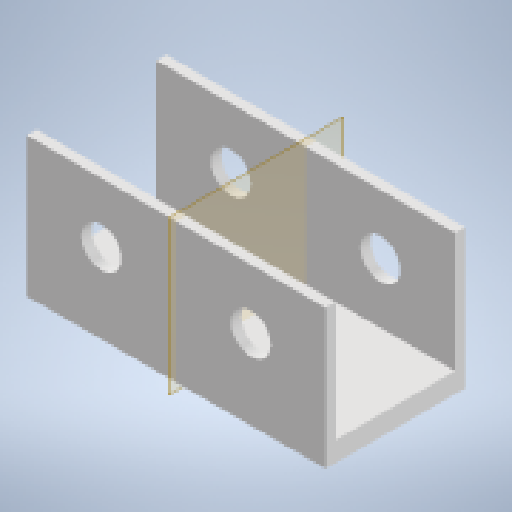
# Autodesk Inventor part: baza
Saved by Autodesk Inventor 2025 (Build 290162000, 162)
## iProperties
Created: 2025-02-05
Part Number: baza
Material: Generic
Document SubType Name: Modeling
Designer: piotr
Density: 1 g/cm^3
Appearance: Default
Author: piotr
Autodesk Inventor part; units mm, degrees
ref_plane "YZ Plane" through (0, 0, 0) normal (1, 0, 0) x (0, 1, 0)
ref_plane "XZ Plane" through (0, 0, 0) normal (0, 1, 0) x (-1, 0, 0)
ref_plane "XY Plane" through (0, 0, 0) normal (0, 0, 1) x (1, 0, 0)
sketch "Sketch1" plane through (0, 0, 0) normal (1, 0, 0) x (0, 1, 0)
  line L0 (0, 0) -> (0, -70)
  line L1 (0, 0) -> (70, 0)
  line L2 (70, 0) -> (70, -5)
  line L3 (70, -5) -> (10, -5)
  line L4 (10, -5) -> (10, -65)
  line L5 (10, -65) -> (70, -65)
  line L6 (70, -65) -> (70, -70)
  line L7 (70, -70) -> (0, -70)
  dimension "d0" = 70
  dimension "d1" = 70
  dimension "d2" = 5
  dimension "d3" = 60
  dimension "d4" = 60
  dimension "d5" = 60
  dimension "d6" = 5
  constraints: 16 end point, 3 horizontal, 3 perpendicular, 2 vertical, 1 point on line
  measures "d0" distance of L0.start L0.end
  measures "d1" distance of L0.start L1.end
  measures "d2" distance of L1.end L2.end
  measures "d3" distance of L2.end L3.end
  measures "d4" distance of L3.end L4.end
  measures "d5" distance of L4.end L5.end
  measures "d6" distance of L5.end L6.end
extrude "Extrusion1" add sketch "Sketch1" along normal blind 150
sketch "Sketch2" plane through (0, 0, 0) normal (0, 0, 1) x (1, 0, 0)
  line L0 (0, 0) -> (0, 70) projected
  line L1 (150, 70) -> (150, 0) projected
  line L2 (0, 10) -> (150, 10) projected
  line L3 (0, 70) -> (150, 70) projected
  line L4 (75, 70) -> (75, 10)
  line L5 (150, 10) -> (150, 70) projected
  line L6 (75, 70) -> (150, 10)
  line L7 (150, 70) -> (75, 10)
  circle A0 centre (112.5, 40) radius 10
  dimension "d9" = 150
  dimension "d10" = 20
  constraints: 6 end point, 3 midpoint, 1 centre point
  measures "d9" distance between parallel lines of L1 L0
  measures "d10" diameter of A0
extrude "Extrusion2" cut sketch "Sketch2" against normal blind 150 contours A0 L6 L7 | L7 L6 A0 | A0 L7 L6 | L6 L7 A0
ref_plane "Work Plane1" through (75, 0, 0) normal (1, 0, 0) x (0, 0, -1)
mirror "Mirror1" about plane through (75, 0, 0) normal (1, 0, 0) of "Extrusion2"
body "Solid1"
